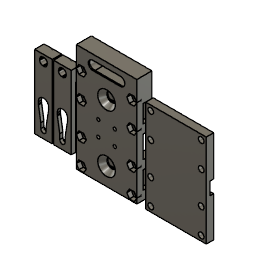
tool change neck (Autodesk Fusion 360 design; units mm, degrees)
Autodesk Fusion 360 part; units mm, degrees
note: some values were not read from the file. Set by a fixed rule: which sketch regions a step uses.
sketch "Sketch1" plane through (0, 0, 0) normal (0, 0, 1) x (1, 0, 0)
  line L0 (24, 8.75) -> (-24, 8.75)
  line L1 (-24, 8.75) -> (-24, -8.75)
  line L2 (-24, -8.75) -> (24, -8.75)
  line L3 (24, -8.75) -> (24, 8.75)
  line L4 (24, 8.75) -> (-24, -8.75) construction
  line L5 (-24, 8.75) -> (24, -8.75) construction
  line L6 (6.5, 6) -> (-6.5, 6)
  line L7 (-6.5, 6) -> (-6.5, -6)
  line L8 (-6.5, -6) -> (6.5, -6)
  line L9 (6.5, -6) -> (6.5, 6)
  line L10 (6.5, 6) -> (-6.5, -6) construction
  line L11 (-6.5, 6) -> (6.5, -6) construction
  circle A0 centre (6.5, 6) radius 1.25
  circle A1 centre (6.5, -6) radius 1.25
  circle A2 centre (-6.5, -6) radius 1.25
  circle A3 centre (-6.5, 6) radius 1.25
  line L12 (24, 36.75) -> (-24, 36.75)
  line L13 (-24, 36.75) -> (-24, -36.75)
  line L14 (-24, -36.75) -> (24, -36.75)
  line L15 (24, -36.75) -> (24, 36.75)
  line L16 (24, 36.75) -> (-24, -36.75) construction
  line L17 (-24, 36.75) -> (24, -36.75) construction
  circle A4 centre (6.5, 6) radius 3
  circle A5 centre (6.5, -6) radius 3
  circle A6 centre (-6.5, -6) radius 3
  circle A7 centre (-6.5, 6) radius 3
  line L18 (0, 36.75) -> (0, 22.75)
  circle A8 centre (0, 22.75) radius 4
  line L19 (0, -36.75) -> (0, -22.75)
  circle A9 centre (0, -22.75) radius 4
  line L20 (24, 36.75) -> (20, 36.75)
  line L21 (20, 36.75) -> (20, 32.75)
  line L22 (20, 32.75) -> (24, 32.75)
  line L23 (24, 32.75) -> (24, 36.75)
  line L24 (-24, 36.75) -> (-20, 36.75)
  line L25 (-20, 36.75) -> (-20, 32.75)
  line L26 (-20, 32.75) -> (-24, 32.75)
  line L27 (-24, 32.75) -> (-24, 36.75)
  line L28 (24, -36.75) -> (20, -36.75)
  line L29 (20, -36.75) -> (20, -32.75)
  line L30 (20, -32.75) -> (24, -32.75)
  line L31 (24, -32.75) -> (24, -36.75)
  line L32 (-24, -36.75) -> (-20, -36.75)
  line L33 (-20, -36.75) -> (-20, -32.75)
  line L34 (-20, -32.75) -> (-24, -32.75)
  line L35 (-24, -32.75) -> (-24, -36.75)
  circle A10 centre (-20, -32.75) radius 0.95
  circle A11 centre (20, -32.75) radius 0.95
  circle A12 centre (20, 32.75) radius 0.95
  circle A13 centre (-20, 32.75) radius 0.95
  circle A14 centre (-20, 32.75) radius 1.85
  circle A15 centre (20, 32.75) radius 1.85
  circle A16 centre (-20, -32.75) radius 1.85
  circle A17 centre (20, -32.75) radius 1.85
  line L36 (24, 8.75) -> (20, 8.75)
  line L37 (20, 8.75) -> (20, 12.75)
  line L38 (20, 12.75) -> (24, 12.75)
  line L39 (24, 12.75) -> (24, 8.75)
  line L40 (-24, 8.75) -> (-20, 8.75)
  line L41 (-20, 8.75) -> (-20, 12.75)
  line L42 (-20, 12.75) -> (-24, 12.75)
  line L43 (-24, 12.75) -> (-24, 8.75)
  line L44 (-24, -8.75) -> (-20, -8.75)
  line L45 (-20, -8.75) -> (-20, -12.75)
  line L46 (-20, -12.75) -> (-24, -12.75)
  line L47 (-24, -12.75) -> (-24, -8.75)
  line L48 (24, -8.75) -> (20, -8.75)
  line L49 (20, -8.75) -> (20, -12.75)
  line L50 (20, -12.75) -> (24, -12.75)
  line L51 (24, -12.75) -> (24, -8.75)
  circle A18 centre (-20, -12.75) radius 1.85
  circle A19 centre (20, -12.75) radius 1.85
  circle A20 centre (-20, 12.75) radius 1.85
  circle A21 centre (20, 12.75) radius 1.85
  line L52 (-24, 36.75) -> (-24, 22.75)
  line L53 (-24, 22.75) -> (-4, 22.75)
  line L54 (-24, -36.75) -> (-24, -22.75)
  line L55 (-24, -22.75) -> (-4, -22.75)
  circle A22 centre (-14, -22.75) radius 1.9
  circle A23 centre (-14, 22.75) radius 1.9
  line L56 (99, -36.75) -> (51, -36.75)
  line L57 (51, -36.75) -> (51, 36.75)
  line L58 (51, 36.75) -> (99, 36.75)
  line L59 (99, 36.75) -> (99, -36.75)
  line L60 (99, -36.75) -> (51, 36.75) construction
  line L61 (51, -36.75) -> (99, 36.75) construction
  line L62 (99, -8.75) -> (51, -8.75)
  line L63 (51, -8.75) -> (51, 8.75)
  line L64 (51, 8.75) -> (99, 8.75)
  line L65 (99, 8.75) -> (99, -8.75)
  line L66 (99, -8.75) -> (51, 8.75) construction
  line L67 (51, -8.75) -> (99, 8.75) construction
  line L68 (51, 36.75) -> (55, 36.75)
  line L69 (55, 36.75) -> (55, 32.75)
  line L70 (55, 32.75) -> (51, 32.75)
  line L71 (51, 32.75) -> (51, 36.75)
  line L72 (99, 36.75) -> (95, 36.75)
  line L73 (95, 36.75) -> (95, 32.75)
  line L74 (95, 32.75) -> (99, 32.75)
  line L75 (99, 32.75) -> (99, 36.75)
  line L76 (51, -36.75) -> (55, -36.75)
  line L77 (55, -36.75) -> (55, -32.75)
  line L78 (55, -32.75) -> (51, -32.75)
  line L79 (51, -32.75) -> (51, -36.75)
  line L80 (99, -36.75) -> (95, -36.75)
  line L81 (95, -36.75) -> (95, -32.75)
  line L82 (95, -32.75) -> (99, -32.75)
  line L83 (99, -32.75) -> (99, -36.75)
  circle A24 centre (55, 32.75) radius 2.25
  circle A25 centre (95, 32.75) radius 2.25
  circle A26 centre (55, -32.75) radius 2.25
  circle A27 centre (95, -32.75) radius 2.25
  line L84 (51, 8.75) -> (55, 8.75)
  line L85 (55, 8.75) -> (55, 12.75)
  line L86 (55, 12.75) -> (51, 12.75)
  line L87 (51, 12.75) -> (51, 8.75)
  circle A28 centre (55, 12.75) radius 2.25
  line L88 (99, 8.75) -> (95, 8.75)
  line L89 (95, 8.75) -> (95, 12.75)
  line L90 (95, 12.75) -> (99, 12.75)
  line L91 (99, 12.75) -> (99, 8.75)
  circle A29 centre (95, 12.75) radius 2.25
  line L92 (51, -8.75) -> (55, -8.75)
  line L93 (55, -8.75) -> (55, -12.75)
  line L94 (55, -12.75) -> (51, -12.75)
  line L95 (51, -12.75) -> (51, -8.75)
  line L96 (99, -8.75) -> (95, -8.75)
  line L97 (95, -8.75) -> (95, -12.75)
  line L98 (95, -12.75) -> (99, -12.75)
  line L99 (99, -12.75) -> (99, -8.75)
  circle A30 centre (55, -12.75) radius 2.25
  circle A31 centre (95, -12.75) radius 2.25
  line L100 (99, 5) -> (51, 5)
  line L101 (51, 5) -> (51, -5)
  line L102 (51, -5) -> (99, -5)
  line L103 (99, -5) -> (99, 5)
  line L104 (99, 5) -> (51, -5) construction
  line L105 (51, 5) -> (99, -5) construction
  line L106 (-43, -29) -> (-57, -29)
  line L107 (-57, -29) -> (-57, 29)
  line L108 (-57, 29) -> (-43, 29)
  line L109 (-43, 29) -> (-43, -29)
  line L110 (-43, -29) -> (-57, 29) construction
  line L111 (-57, -29) -> (-43, 29) construction
  line L112 (-57, 29) -> (-43, 29)
  line L113 (-43, 29) -> (-43, 19)
  line L114 (-43, 19) -> (-57, 19)
  line L115 (-57, 19) -> (-57, 29)
  line L116 (-43, 19) -> (-43, 21.5068)
  line L117 (-43, 21.5068) -> (-43, 29)
  line L118 (-44, 29) -> (-44, 29)
  line L119 (-43, 29) -> (-43, 19)
  line L120 (-43, 29) -> (-50, 29)
  line L121 (-50, 29) -> (-50, 24)
  line L122 (-50, 24) -> (-43, 24)
  line L123 (-43, 24) -> (-43, 29)
  line L124 (-47, 27) -> (-53, 27)
  line L125 (-53, 27) -> (-53, 21)
  line L126 (-53, 21) -> (-47, 21)
  line L127 (-47, 21) -> (-47, 27)
  line L128 (-47, 27) -> (-53, 21) construction
  line L129 (-53, 27) -> (-47, 21) construction
  line L130 (-50, 24) -> (-50, -5)
  circle A32 centre (-50, -5) radius 4
  line L131 (-50, -5) -> (-50, -7)
  line L132 (-50, -7) -> (-50, -19)
  circle A33 centre (-50, -7) radius 4
  line L133 (-46.0119, -4.6913) -> (-46.0001, -6.9792)
  line L134 (-53.9727, -5.4669) -> (-53.9993, -6.9269)
  circle A34 centre (-50, -19) radius 2.1
  line L135 (-50, -19) -> (-50, -23)
  circle A35 centre (-50, -23) radius 2.1
  line L136 (-47.9, -19) -> (-47.9, -23)
  line L137 (-52.1, -23) -> (-52.1, -19)
  line L138 (-47.9, -19) -> (-46.0519, -7.6424)
  line L139 (-52.1, -19) -> (-53.9481, -7.6424)
  line L140 (-24, 36.75) -> (24, 36.75)
  line L141 (24, 36.75) -> (24, 46.75)
  line L142 (24, 46.75) -> (-24, 46.75)
  line L143 (-24, 46.75) -> (-24, 36.75)
  line L144 (51, 36.75) -> (99, 36.75)
  line L145 (99, 36.75) -> (99, 46.75)
  line L146 (99, 46.75) -> (51, 46.75)
  line L147 (51, 46.75) -> (51, 36.75)
  line L148 (51, 46.75) -> (55, 46.75)
  line L149 (55, 46.75) -> (55, 42.75)
  line L150 (55, 42.75) -> (51, 42.75)
  line L151 (51, 42.75) -> (51, 46.75)
  line L152 (99, 46.75) -> (95, 46.75)
  line L153 (95, 46.75) -> (95, 42.75)
  line L154 (95, 42.75) -> (99, 42.75)
  line L155 (99, 42.75) -> (99, 46.75)
  circle A36 centre (95, 42.75) radius 2.25
  circle A37 centre (55, 42.75) radius 2.25
  line L156 (24, 46.75) -> (20, 46.75)
  line L157 (20, 46.75) -> (20, 42.75)
  line L158 (20, 42.75) -> (24, 42.75)
  line L159 (24, 42.75) -> (24, 46.75)
  line L160 (-24, 46.75) -> (-20, 46.75)
  line L161 (-20, 46.75) -> (-20, 42.75)
  line L162 (-20, 42.75) -> (-24, 42.75)
  line L163 (-24, 42.75) -> (-24, 46.75)
  circle A38 centre (20, 42.75) radius 1.85
  circle A39 centre (-20, 42.75) radius 1.85
  line L164 (21.963, 29.35) -> (23.926, 32.75)
  line L165 (23.926, 32.75) -> (21.963, 36.15)
  line L166 (21.963, 36.15) -> (18.037, 36.15)
  line L167 (18.037, 36.15) -> (16.074, 32.75)
  line L168 (16.074, 32.75) -> (18.037, 29.35)
  line L169 (18.037, 29.35) -> (21.963, 29.35)
  line L170 (-18.037, 29.35) -> (-16.074, 32.75)
  line L171 (-16.074, 32.75) -> (-18.037, 36.15)
  line L172 (-18.037, 36.15) -> (-21.963, 36.15)
  line L173 (-21.963, 36.15) -> (-23.926, 32.75)
  line L174 (-23.926, 32.75) -> (-21.963, 29.35)
  line L175 (-21.963, 29.35) -> (-18.037, 29.35)
  line L176 (21.963, -36.15) -> (23.926, -32.75)
  line L177 (23.926, -32.75) -> (21.963, -29.35)
  line L178 (21.963, -29.35) -> (18.037, -29.35)
  line L179 (18.037, -29.35) -> (16.074, -32.75)
  line L180 (16.074, -32.75) -> (18.037, -36.15)
  line L181 (18.037, -36.15) -> (21.963, -36.15)
  line L182 (-18.037, -36.15) -> (-16.074, -32.75)
  line L183 (-16.074, -32.75) -> (-18.037, -29.35)
  line L184 (-18.037, -29.35) -> (-21.963, -29.35)
  line L185 (-21.963, -29.35) -> (-23.926, -32.75)
  line L186 (-23.926, -32.75) -> (-21.963, -36.15)
  line L187 (-21.963, -36.15) -> (-18.037, -36.15)
  line L188 (21.963, 9.35) -> (23.926, 12.75)
  line L189 (23.926, 12.75) -> (21.963, 16.15)
  line L190 (21.963, 16.15) -> (18.037, 16.15)
  line L191 (18.037, 16.15) -> (16.074, 12.75)
  line L192 (16.074, 12.75) -> (18.037, 9.35)
  line L193 (18.037, 9.35) -> (21.963, 9.35)
  line L194 (21.963, -16.15) -> (23.926, -12.75)
  line L195 (23.926, -12.75) -> (21.963, -9.35)
  line L196 (21.963, -9.35) -> (18.037, -9.35)
  line L197 (18.037, -9.35) -> (16.074, -12.75)
  line L198 (16.074, -12.75) -> (18.037, -16.15)
  line L199 (18.037, -16.15) -> (21.963, -16.15)
  line L200 (-18.037, 9.35) -> (-16.074, 12.75)
  line L201 (-16.074, 12.75) -> (-18.037, 16.15)
  line L202 (-18.037, 16.15) -> (-21.963, 16.15)
  line L203 (-21.963, 16.15) -> (-23.926, 12.75)
  line L204 (-23.926, 12.75) -> (-21.963, 9.35)
  line L205 (-21.963, 9.35) -> (-18.037, 9.35)
  line L206 (-18.037, -16.15) -> (-16.074, -12.75)
  line L207 (-16.074, -12.75) -> (-18.037, -9.35)
  line L208 (-18.037, -9.35) -> (-21.963, -9.35)
  line L209 (-21.963, -9.35) -> (-23.926, -12.75)
  line L210 (-23.926, -12.75) -> (-21.963, -16.15)
  line L211 (-21.963, -16.15) -> (-18.037, -16.15)
  point P0 (75, 0)
  point P1 (75, 0)
  point P2 (75, 0)
  point P3 (-50, 0)
  point P4 (-50, 24)
  point P5 (20, 32.75)
  point P6 (-20, 32.75)
  point P7 (20, -32.75)
  point P8 (-20, -32.75)
  point P9 (20, 12.75)
  point P10 (20, -12.75)
  point P11 (-20, 12.75)
  point P12 (-20, -12.75)
  dimension "d1" = 48
  dimension "d2" = 17.5
  dimension "d3" = 13
  dimension "d4" = 12
  dimension "d5" = 2.5
  dimension "d6" = 2.5
  dimension "d7" = 2.5
  dimension "d8" = 2.5
  dimension "d11" = 48
  dimension "d12" = 73.5
  dimension "d30" = 6
  dimension "d31" = 6
  dimension "d32" = 6
  dimension "d33" = 6
  dimension "d38" = 14
  dimension "d39" = 8
  dimension "d40" = 14
  dimension "d41" = 8
  dimension "d50" = 4
  dimension "d51" = 4
  dimension "d52" = 4
  dimension "d53" = 4
  dimension "d54" = 4
  dimension "d55" = 4
  dimension "d56" = 4
  dimension "d57" = 4
  dimension "d58" = 1.9
  dimension "d59" = 1.9
  dimension "d60" = 1.9
  dimension "d61" = 1.9
  dimension "d62" = 3.7
  dimension "d63" = 3.7
  dimension "d64" = 3.7
  dimension "d65" = 3.7
  dimension "d86" = 4
  dimension "d87" = 4
  dimension "d88" = 4
  dimension "d89" = 4
  dimension "d90" = 4
  dimension "d91" = 4
  dimension "d92" = 4
  dimension "d93" = 4
  dimension "d94" = 3.7
  dimension "d95" = 3.7
  dimension "d96" = 3.7
  dimension "d97" = 3.7
  dimension "d114" = 14
  dimension "d115" = 14
  dimension "d116" = 3.8
  dimension "d117" = 3.8
  dimension "d118" = 48
  dimension "d119" = 73.5
  dimension "d120" = 48
  dimension "d121" = 17.5
  dimension "d122" = 4
  dimension "d123" = 4
  dimension "d124" = 4
  dimension "d125" = 4
  dimension "d126" = 4
  dimension "d127" = 4
  dimension "d128" = 4
  dimension "d129" = 4
  dimension "d130" = 4.5
  dimension "d131" = 4.5
  dimension "d132" = 4.5
  dimension "d133" = 4.5
  dimension "d136" = 4
  dimension "d137" = 4
  dimension "d138" = 4.5
  dimension "d139" = 4
  dimension "d140" = 4
  dimension "d141" = 4.5
  dimension "d142" = 4
  dimension "d143" = 4
  dimension "d144" = 4
  dimension "d145" = 4
  dimension "d146" = 4.5
  dimension "d147" = 4.5
  dimension "d148" = 48
  dimension "d149" = 10
  dimension "d154" = 14
  dimension "d155" = 58
  dimension "d156" = 14
  dimension "d157" = 10
  dimension "d158" = 7
  dimension "d159" = 5
  dimension "d160" = 6
  dimension "d161" = 6
  dimension "d162" = 29
  dimension "d163" = 8
  dimension "d164" = 2
  dimension "d165" = 12
  dimension "d166" = 8
  dimension "d167" = 4.2
  dimension "d168" = 4
  dimension "d169" = 4.2
  dimension "d211" = 10
  dimension "d212" = 48
  dimension "d213" = 10
  dimension "d214" = 4
  dimension "d215" = 4
  dimension "d216" = 4
  dimension "d217" = 4
  dimension "d218" = 4.5
  dimension "d219" = 4.5
  dimension "d220" = 4
  dimension "d221" = 4
  dimension "d222" = 4
  dimension "d223" = 4
  dimension "d224" = 3.7
  dimension "d225" = 3.7
  dimension "d254" = 3.4
  dimension "d255" = 3.4
  dimension "d256" = 3.4
  dimension "d257" = 3.4
  dimension "d262" = 3.4
  dimension "d263" = 3.4
  dimension "d264" = 3.4
  dimension "d265" = 3.4
  constraint horizontal L0
  constraint perpendicular L0 L1
  constraint parallel L0 L2
  constraint parallel L1 L3
  constraint coincident L4 origin
  constraint coincident L5 origin
  constraint horizontal L6
  constraint perpendicular L6 L7
  constraint parallel L6 L8
  constraint parallel L7 L9
  constraint coincident L10 origin
  constraint coincident L11 origin
  constraint coincident L6.start L9.end
  constraint coincident L8.end L9.start
  constraint coincident L7.end L8.start
  constraint coincident L6.end L7.start
  constraint horizontal L12
  constraint perpendicular L12 L13
  constraint parallel L12 L14
  constraint parallel L13 L15
  constraint coincident L16 origin
  constraint coincident L17 origin
  constraint concentric A0 A4
  constraint concentric A1 A5
  constraint concentric A2 A6
  constraint concentric A3 A7
  constraint midpoint L12 L18.start
  constraint perpendicular L12 L18
  constraint coincident L18.end A8.centre
  constraint midpoint L14 L19.start
  constraint perpendicular L14 L19
  constraint coincident L19.end A9.centre
  constraint horizontal L20
  constraint vertical L21
  constraint horizontal L22
  constraint vertical L23
  constraint horizontal L24
  constraint vertical L25
  constraint horizontal L26
  constraint vertical L27
  constraint horizontal L28
  constraint vertical L29
  constraint horizontal L30
  constraint vertical L31
  constraint horizontal L32
  constraint vertical L33
  constraint horizontal L34
  constraint vertical L35
  constraint coincident P8 L33.end
  constraint coincident P7 L29.end
  constraint coincident P5 L21.end
  constraint coincident P6 L25.end
  constraint concentric A13 A14
  constraint concentric A10 A16
  constraint concentric A11 A17
  constraint horizontal L36
  constraint vertical L37
  constraint horizontal L38
  constraint vertical L39
  constraint horizontal L40
  constraint vertical L41
  constraint horizontal L42
  constraint vertical L43
  constraint horizontal L44
  constraint vertical L45
  constraint horizontal L46
  constraint vertical L47
  constraint horizontal L48
  constraint vertical L49
  constraint horizontal L50
  constraint vertical L51
  constraint coincident P12 L45.end
  constraint coincident P10 L49.end
  constraint coincident P11 L41.end
  constraint coincident P9 L37.end
  constraint perpendicular L26 L52
  constraint coincident A8 L53.end
  constraint perpendicular L52 L53
  constraint perpendicular L14 L54
  constraint coincident A9 L55.end
  constraint perpendicular L54 L55
  constraint midpoint L55 A22.centre
  constraint midpoint L53 A23.centre
  constraint horizontal L56
  constraint perpendicular L56 L57
  constraint parallel L56 L58
  constraint parallel L57 L59
  constraint coincident L60 P2
  constraint coincident L61 P2
  constraint horizontal L62
  constraint perpendicular L62 L63
  constraint parallel L62 L64
  constraint parallel L63 L65
  constraint coincident L66 P2
  constraint coincident L67 P2
  constraint coincident P2 P1
  constraint horizontal L68
  constraint vertical L69
  constraint horizontal L70
  constraint vertical L71
  constraint horizontal L72
  constraint vertical L73
  constraint horizontal L74
  constraint vertical L75
  constraint horizontal L76
  constraint vertical L77
  constraint horizontal L78
  constraint vertical L79
  constraint horizontal L80
  constraint vertical L81
  constraint horizontal L82
  constraint vertical L83
  constraint coincident L69.end L70.start
  constraint coincident L73.end L74.start
  constraint coincident L77.end L78.start
  constraint coincident L81.end L82.start
  constraint horizontal L84
  constraint vertical L85
  constraint horizontal L86
  constraint vertical L87
  constraint coincident L85.end L86.start
  constraint horizontal L88
  constraint vertical L89
  constraint horizontal L90
  constraint vertical L91
  constraint coincident L89.end L90.start
  constraint horizontal L92
  constraint vertical L93
  constraint horizontal L94
  constraint vertical L95
  constraint horizontal L96
  constraint vertical L97
  constraint horizontal L98
  constraint vertical L99
  constraint coincident L93.end L94.start
  constraint coincident L97.end L98.start
  constraint horizontal L100
  constraint perpendicular L100 L101
  constraint parallel L100 L102
  constraint parallel L101 L103
  constraint coincident L104 P2
  constraint coincident L105 P2
  constraint horizontal L106
  constraint perpendicular L106 L107
  constraint parallel L106 L108
  constraint parallel L107 L109
  constraint coincident L110 P3
  constraint coincident L111 P3
  constraint horizontal L112
  constraint vertical L113
  constraint horizontal L114
  constraint vertical L115
  constraint vertical L117
  constraint vertical L119
  constraint coincident L113 L108.end
  constraint horizontal L120
  constraint vertical L121
  constraint horizontal L122
  constraint vertical L123
  constraint horizontal L124
  constraint perpendicular L124 L125
  constraint parallel L124 L126
  constraint parallel L125 L127
  constraint coincident L128 P4
  constraint coincident L129 P4
  constraint coincident P4 L121.end
  constraint perpendicular L114 L130
  constraint coincident L130.end A32.centre
  constraint vertical L131
  constraint parallel L131 L132
  constraint coincident L131.end L132.start
  constraint coincident A32 L133.start
  constraint coincident A33 L133.end
  constraint tangent A33 L133
  constraint coincident A32 L134.start
  constraint coincident A33 L134.end
  constraint tangent A33 L134
  constraint coincident L132.end A34.centre
  constraint parallel L132 L135
  constraint coincident L135.end A35.centre
  constraint coincident A34 L136.start
  constraint coincident A35 L136.end
  constraint tangent A35 L136
  constraint parallel L132 L136
  constraint coincident A35 L137.start
  constraint coincident A34 L137.end
  constraint tangent A34 L137
  constraint vertical L137
  constraint coincident A33 L138.end
  constraint tangent A33 L138
  constraint coincident A33 L139.end
  constraint tangent A33 L139
  constraint horizontal L140
  constraint vertical L141
  constraint horizontal L142
  constraint vertical L143
  constraint horizontal L144
  constraint vertical L145
  constraint horizontal L146
  constraint vertical L147
  constraint horizontal L148
  constraint vertical L149
  constraint horizontal L150
  constraint vertical L151
  constraint horizontal L152
  constraint vertical L153
  constraint horizontal L154
  constraint vertical L155
  constraint coincident L153.end L154.start
  constraint coincident L149.end L150.start
  constraint horizontal L156
  constraint vertical L157
  constraint horizontal L158
  constraint vertical L159
  constraint horizontal L160
  constraint vertical L161
  constraint horizontal L162
  constraint vertical L163
  constraint coincident L157.end L158.start
  constraint coincident L161.end L162.start
  measures "d1" distance of L1.end L2.end
  measures "d2" distance of L0.end L1.end
  measures "d3" distance of L7.end L8.end
  measures "d4" distance of L6.end L7.end
  measures "d5" diameter of A0
  measures "d6" diameter of A1
  measures "d7" diameter of A2
  measures "d8" diameter of A3
  measures "d11" distance of L13.end L14.end
  measures "d12" distance of L12.end L13.end
  measures "d30" diameter of A4
  measures "d31" diameter of A5
  measures "d32" diameter of A6
  measures "d33" diameter of A7
  measures "d38" distance of L18.start L18.end
  measures "d39" diameter of A8
  measures "d40" distance of L19.start L19.end
  measures "d41" diameter of A9
  measures "d50" distance of L12.start L20.end
  measures "d51" distance of L12.start L22.end
  measures "d52" distance of L12.end L24.end
  measures "d53" distance of L12.end L26.end
  measures "d54" distance of L14.end L28.end
  measures "d55" distance of L14.end L30.end
  measures "d56" distance of L13.end L32.end
  measures "d57" distance of L13.end L34.end
  measures "d58" diameter of A10
  measures "d59" diameter of A11
  measures "d60" diameter of A12
  measures "d61" diameter of A13
  measures "d62" diameter of A14
  measures "d63" diameter of A15
  measures "d64" diameter of A16
  measures "d65" diameter of A17
  measures "d86" distance of L0.start L36.end
  measures "d87" distance of L0.start L38.end
  measures "d88" distance of L0.end L40.end
  measures "d89" distance of L0.end L42.end
  measures "d90" distance of L1.end L44.end
  measures "d91" distance of L1.end L46.end
  measures "d92" distance of L2.end L48.end
  measures "d93" distance of L2.end L50.end
  measures "d94" diameter of A18
  measures "d95" diameter of A19
  measures "d96" diameter of A20
  measures "d97" diameter of A21
  measures "d114" distance of L12.end L52.end
  measures "d115" distance of L13.end L54.end
  measures "d116" diameter of A22
  measures "d117" diameter of A23
  measures "d118" distance of L57.end L58.end
  measures "d119" distance of L56.end L57.end
  measures "d120" distance of L63.end L64.end
  measures "d121" distance of L62.end L63.end
  measures "d122" distance of L57.end L68.end
  measures "d123" distance of L57.end L70.end
  measures "d124" distance of L58.end L72.end
  measures "d125" distance of L58.end L74.end
  measures "d126" distance of L56.end L76.end
  measures "d127" distance of L56.end L78.end
  measures "d128" distance of L56.start L80.end
  measures "d129" distance of L56.start L82.end
  measures "d130" diameter of A24
  measures "d131" diameter of A25
  measures "d132" diameter of A26
  measures "d133" diameter of A27
  measures "d136" distance of L63.end L84.end
  measures "d137" distance of L63.end L86.end
  measures "d138" diameter of A28 A4
  measures "d139" distance of L64.end L88.end
  measures "d140" distance of L64.end L90.end
  measures "d141" diameter of A29
  measures "d142" distance of L62.end L92.end
  measures "d143" distance of L62.end L94.end
  measures "d144" distance of L62.start L96.end
  measures "d145" distance of L62.start L98.end
  measures "d146" diameter of A30
  measures "d147" diameter of A31
  measures "d148" distance of L101.end L102.end
  measures "d149" distance of L100.end L101.end
  measures "d154" distance of L107.end L108.end
  measures "d155" distance of L106.end L107.end
  measures "d156" distance of L107.end L108.end
  measures "d157" distance of L107.end L114.end
  measures "d158" distance of L108.end L120.end
  measures "d159" distance of L108.end L122.end
  measures "d160" distance of L125.end L126.end
  measures "d161" distance of L124.end L125.end
  measures "d162" distance of P4 L130.end
  measures "d163" diameter of A32
  measures "d164" distance of L130.end L131.end
  measures "d165" distance of L131.end L132.end
  measures "d166" diameter of A33
  measures "d167" diameter of A34
  measures "d168" distance of L132.end L135.end
  measures "d169" diameter of A35
  measures "d211" distance of L12.end L142.end
  measures "d212" distance of L57.end L58.end
  measures "d213" distance of L57.end L146.end
  measures "d214" distance of L146.end L148.end
  measures "d215" distance of L146.end L150.end
  measures "d216" distance of L145.end L152.end
  measures "d217" distance of L145.end L154.end
  measures "d219" diameter of A37 A4
  measures "d220" distance of L141.end L156.end
  measures "d221" distance of L141.end L158.end
  measures "d222" distance of L142.end L160.end
  measures "d223" distance of L142.end L162.end
  measures "d224" diameter of A38
  measures "d225" diameter of A39
  measures "d254" distance of P5 L169
  measures "d255" distance of P6 L175
  measures "d256" distance of P7 L181
  measures "d257" distance of P8 L187
  measures "d262" distance of P9 L193
  measures "d263" distance of P10 L199
  measures "d264" distance of P11 L205
  measures "d265" distance of P12 L211
extrude "Extrude1" add sketch "Sketch1" along normal blind 12 contours L0 L2 L3 L9 L15 A4 A5 L36 L48 | L0 L15 L36 L37 L38 L39 L188 L193 | L0 L12 L13 L15 A4 A7 L18 A8 L21 L22 L37 L38 L41 L42 L53 A23 L140 L164 L166 L167 L168 L169 L189 L190 L191 L192 L193 L200 L201 L202 L203 L205 | L2 L15 L48 L49 L50 L51 L195 L196 | L0 L6 L9 A0 A4 | L0 A4 | L37 L38 A21 L189 L190 L191 L192 L193 | L37 L38 A21 L188 L193 | L2 L13 L14 L15 A5 A6 L19 A9 L29 L30 L45 L46 L49 L50 L55 A22 L177 L178 L179 L180 L181 L194 L196 L197 L198 L199 L206 L207 L208 L210 L211 | L12 L15 L20 L21 L22 L23 L140 L165 L166 | L0 L6 A4 A7 | L2 A5 | L2 L8 L9 A1 A5 | L49 L50 A19 L195 L196 | L49 L50 A19 L194 L196 L197 L198 L199 | L14 L15 L28 L29 L30 L31 L176 L181 | L21 L22 A15 L164 L166 L167 L168 L169 | L21 L22 A15 L165 L166 | L0 L6 L7 A3 A7 | L0 A7 | L6 L7 L8 L9 A4 A5 A6 A7 | L6 L9 A0 A4 | L2 L8 A5 A6 | L29 L30 A17 L176 L181 | L29 L30 A17 L177 L178 L179 L180 L181 | L0 L1 L2 L7 L13 A6 A7 L40 L44 | L6 L7 A3 A7 | L8 L9 A1 A5 | L2 A6 | L2 L7 L8 A2 A6 | L12 L13 L18 A8 L25 L26 L52 L53 A23 L140 L170 L171 L172 L174 L175 | L0 L13 L40 L41 L42 L43 L204 L205 | L7 L8 A2 A6 | L13 L14 L19 A9 L33 L34 L54 L55 A22 L182 L183 L184 L185 L187 | L12 L13 L24 L25 L26 L27 L52 L140 L172 L173 | A8 | L41 L42 A20 L204 L205 | L41 L42 A20 L200 L201 L202 L203 L205 | L2 L13 L44 L45 L46 L47 L208 L209 | L13 L14 L32 L33 L34 L35 L54 L186 L187 | A9 | L25 L26 A14 L170 L171 L172 L174 L175 | L25 L26 A14 L172 L173 | L45 L46 A18 L206 L207 L208 L210 L211 | L45 L46 A18 L208 L209 | L33 L34 A16 L186 L187 | L33 L34 A16 L182 L183 L184 L185 L187 | L53 A23 | L53 A23 | L55 A22 | L55 A22 makes body 1
extrude "Extrude2" cut sketch "Sketch1" along normal blind 7 contours L0 L2 L3 L9 L15 A4 A5 L36 L48 | L0 L6 L9 A0 A4 | L0 L6 A4 A7 | L2 L8 L9 A1 A5 | L0 L6 L7 A3 A7 | L6 L7 L8 L9 A4 A5 A6 A7 | L6 L9 A0 A4 | L2 L8 A5 A6 | L0 L1 L2 L7 L13 A6 A7 L40 L44 | L6 L7 A3 A7 | L8 L9 A1 A5 | L2 L7 L8 A2 A6 | L7 L8 A2 A6 bodies 1
extrude "Extrude3" cut sketch "Sketch1" along normal blind 19 contours A8 | A9 bodies 1
extrude "Extrude19" cut sketch "Sketch1" along normal blind 12 and the other way blind -8.5 contours L37 L38 A21 L189 L190 L191 L192 L193 | L37 L38 A21 L188 L193 | L49 L50 A19 L195 L196 | L49 L50 A19 L194 L196 L197 L198 L199 | L21 L22 A15 L164 L166 L167 L168 L169 | L21 L22 A15 L165 L166 | L29 L30 A17 L176 L181 | L29 L30 A17 L177 L178 L179 L180 L181 | L41 L42 A20 L204 L205 | L41 L42 A20 L200 L201 L202 L203 L205 | L25 L26 A14 L170 L171 L172 L174 L175 | L25 L26 A14 L172 L173 | L45 L46 A18 L206 L207 L208 L210 L211 | L45 L46 A18 L208 L209 | L33 L34 A16 L186 L187 | L33 L34 A16 L182 L183 L184 L185 L187 bodies 1
sketch "Sketch3" plane through (24, 0, 0) normal (1, 0, 0) x (0, 0, -1)
  line L0 (0, 8.75) -> (0, 36.75)
  line L1 (-12, 36.75) -> (-12, -36.75)
  line L2 (-12, -36.75) -> (0, -36.75)
  line L3 (-12, 36.75) -> (-7, 36.75)
  line L4 (-7, 36.75) -> (-7, -36.75)
  line L5 (-7, -36.75) -> (-12, -36.75)
  line L6 (-12, -36.75) -> (-12, 36.75)
  line L7 (-7, 36.75) -> (-7, 28.75)
  line L8 (-7, 28.75) -> (-3, 28.75)
  line L9 (-3, 28.75) -> (-3, 16.75)
  line L10 (-3, 16.75) -> (-7, 16.75)
  line L11 (-7, 16.75) -> (-7, 28.75)
  line L12 (-7, -36.75) -> (-7, -28.75)
  line L13 (-7, -28.75) -> (-3, -28.75)
  line L14 (-3, -28.75) -> (-3, -16.75)
  line L15 (-3, -16.75) -> (-7, -16.75)
  line L16 (-7, -16.75) -> (-7, -28.75)
  line L17 (-7, 12.75) -> (-7, 28.75)
  line L18 (-7, -24.75) -> (-7, -16.75)
  line L19 (-7, -24.75) -> (-7, -23.75)
  line L20 (-7, 28.75) -> (-10, 28.75)
  line L21 (-10, 28.75) -> (-10, 16.75)
  line L22 (-10, 16.75) -> (-7, 16.75)
  line L23 (-7, 16.75) -> (-7, 28.75)
  line L24 (-7, 28.75) -> (-9, 28.75)
  line L25 (-9, 28.75) -> (-9, 16.75)
  line L26 (-9, 16.75) -> (-7, 16.75)
  line L27 (-7, 16.75) -> (-7, 28.75)
  line L28 (-9, 28.75) -> (-7, 28.75)
  line L29 (-7, 28.75) -> (-7, 27.75)
  line L30 (-7, 27.75) -> (-9, 27.75)
  line L31 (-9, 27.75) -> (-9, 28.75)
  line L32 (-7, 16.75) -> (-9, 16.75)
  line L33 (-9, 16.75) -> (-9, 17.75)
  line L34 (-9, 17.75) -> (-7, 17.75)
  line L35 (-7, 17.75) -> (-7, 16.75)
  line L36 (-7, -16.75) -> (-10, -16.75)
  line L37 (-10, -16.75) -> (-10, -28.75)
  line L38 (-10, -28.75) -> (-7, -28.75)
  line L39 (-7, -28.75) -> (-7, -16.75)
  line L40 (-7, -16.75) -> (-9, -16.75)
  line L41 (-9, -16.75) -> (-9, -28.75)
  line L42 (-9, -28.75) -> (-7, -28.75)
  line L43 (-7, -28.75) -> (-7, -16.75)
  line L44 (-7, -16.75) -> (-9, -16.75)
  line L45 (-9, -16.75) -> (-9, -17.75)
  line L46 (-9, -17.75) -> (-7, -17.75)
  line L47 (-7, -17.75) -> (-7, -16.75)
  line L48 (-7, -28.75) -> (-9, -28.75)
  line L49 (-9, -28.75) -> (-9, -27.75)
  line L50 (-9, -27.75) -> (-7, -27.75)
  line L51 (-7, -27.75) -> (-7, -28.75)
  line L52 (-3, 28.75) -> (-7, 28.75)
  line L53 (-7, 28.75) -> (-7, 29.75)
  line L54 (-7, 29.75) -> (-3, 29.75)
  line L55 (-3, 29.75) -> (-3, 28.75)
  line L56 (-3, 16.75) -> (-7, 16.75)
  line L57 (-7, 16.75) -> (-7, 15.75)
  line L58 (-7, 15.75) -> (-3, 15.75)
  line L59 (-3, 15.75) -> (-3, 16.75)
  line L60 (-3, -16.75) -> (-7, -16.75)
  line L61 (-7, -16.75) -> (-7, -15.75)
  line L62 (-7, -15.75) -> (-3, -15.75)
  line L63 (-3, -15.75) -> (-3, -16.75)
  line L64 (-3, -28.75) -> (-7, -28.75)
  line L65 (-7, -28.75) -> (-7, -29.75)
  line L66 (-7, -29.75) -> (-3, -29.75)
  line L67 (-3, -29.75) -> (-3, -28.75)
  line L68 (0, 36.75) -> (-12, 36.75)
  line L69 (-7, 8.75) -> (0, 8.75)
  line L70 (0, -36.75) -> (0, -8.75)
  line L71 (0, -8.75) -> (-7, -8.75)
  line L72 (-7, -8.75) -> (-7, 8.75)
  dimension "d42" = 5
  dimension "d43" = 73.5
  dimension "d44" = 8
  dimension "d45" = 4
  dimension "d46" = 12
  dimension "d47" = 8
  dimension "d48" = 4
  dimension "d49" = 12
  dimension "d98" = 3
  dimension "d99" = 12
  dimension "d100" = 2
  dimension "d101" = 12
  dimension "d102" = 2
  dimension "d103" = 1
  dimension "d104" = 2
  dimension "d105" = 1
  dimension "d106" = 3
  dimension "d107" = 12
  dimension "d108" = 2
  dimension "d109" = 12
  dimension "d110" = 2
  dimension "d111" = 1
  dimension "d112" = 2
  dimension "d113" = 1
  dimension "d226" = 4
  dimension "d227" = 1
  dimension "d228" = 4
  dimension "d229" = 1
  dimension "d230" = 4
  dimension "d231" = 1
  dimension "d232" = 4
  dimension "d233" = 1
  constraint horizontal L3
  constraint vertical L4
  constraint horizontal L5
  constraint vertical L6
  constraint coincident L1.start L3.start
  constraint perpendicular L3 L7
  constraint horizontal L8
  constraint vertical L9
  constraint horizontal L10
  constraint vertical L11
  constraint perpendicular L5 L12
  constraint horizontal L13
  constraint vertical L14
  constraint horizontal L15
  constraint vertical L16
  constraint vertical L17
  constraint vertical L18
  constraint horizontal L20
  constraint vertical L21
  constraint horizontal L22
  constraint vertical L23
  constraint horizontal L24
  constraint vertical L25
  constraint horizontal L26
  constraint vertical L27
  constraint horizontal L28
  constraint vertical L29
  constraint horizontal L30
  constraint vertical L31
  constraint horizontal L32
  constraint vertical L33
  constraint horizontal L34
  constraint vertical L35
  constraint horizontal L36
  constraint vertical L37
  constraint horizontal L38
  constraint vertical L39
  constraint horizontal L40
  constraint vertical L41
  constraint horizontal L42
  constraint vertical L43
  constraint horizontal L44
  constraint vertical L45
  constraint horizontal L46
  constraint vertical L47
  constraint horizontal L48
  constraint vertical L49
  constraint horizontal L50
  constraint vertical L51
  constraint horizontal L52
  constraint vertical L53
  constraint horizontal L54
  constraint vertical L55
  constraint horizontal L56
  constraint vertical L57
  constraint horizontal L58
  constraint vertical L59
  constraint horizontal L60
  constraint vertical L61
  constraint horizontal L62
  constraint vertical L63
  constraint horizontal L64
  constraint vertical L65
  constraint horizontal L66
  constraint vertical L67
  measures "d42" distance of L1.start L3.end
  measures "d43" distance of L1.start L1.end
  measures "d44" distance of L3.end L7.end
  measures "d45" distance of L7.end L8.end
  measures "d46" distance of L7.end L10.end
  measures "d47" distance of L4.end L12.end
  measures "d48" distance of L12.end L13.end
  measures "d49" distance of L12.end L15.end
  measures "d98" distance of L7.end L20.end
  measures "d99" distance of L7.end L10.end
  measures "d100" distance of L7.end L24.end
  measures "d101" distance of L7.end L10.end
  measures "d102" distance of L24.end L7.end
  measures "d103" distance of L24.end L30.end
  measures "d104" distance of L10.end L25.end
  measures "d105" distance of L10.end L34.end
  measures "d106" distance of L15.end L36.end
  measures "d107" distance of L15.end L12.end
  measures "d108" distance of L15.end L40.end
  measures "d109" distance of L15.end L12.end
  measures "d110" distance of L15.end L40.end
  measures "d111" distance of L15.end L46.end
  measures "d112" distance of L12.end L41.end
  measures "d113" distance of L12.end L50.end
  measures "d226" distance of L8.end L7.end
  measures "d227" distance of L8.end L54.end
  measures "d228" distance of L9.end L10.end
  measures "d229" distance of L9.end L58.end
  measures "d230" distance of L14.end L15.end
  measures "d231" distance of L14.end L62.end
  measures "d232" distance of L13.end L12.end
  measures "d233" distance of L13.end L66.end
extrude "Extrude4" cut sketch "Sketch3" against normal blind 48 contours L4 L7 L8 L52 L53 L54 L55 | L4 L10 L17 L56 L57 L58 L59 | L4 L15 L60 L61 L62 L63 | L4 L8 L9 L10 L11 L17 L23 L27 L29 L35 L52 L56 | L4 L13 L14 L15 L16 L18 L19 L39 L43 L47 L51 L60 L64 | L4 L12 L13 L64 L65 L66 L67 bodies 1
extrude "Extrude9" add sketch "Sketch1" along normal blind 12 and the other way blind -6 separate body contours L56 L59 L80 L81 L82 L83 A27 | L56 L57 L59 L62 L77 L78 L81 L82 A26 A27 L93 L94 L97 L98 A30 A31 | L56 L57 L76 L77 L78 L79 A26 | L59 L62 L96 L97 L98 L99 A31 | L57 L59 L62 L63 L65 L92 L96 L102 | L57 L59 L63 L65 L100 L101 L102 L103 | L57 L62 L92 L93 L94 L95 A30 | L57 L59 L63 L64 L65 L84 L88 L100 | L59 L64 L88 L89 L90 L91 A29 | L57 L58 L59 L64 L69 L70 L73 L74 A24 A25 L85 L86 A28 L89 L90 A29 L144 | L57 L64 L84 L85 L86 L87 A28 | L58 L59 L72 L73 L74 L75 A25 L144 | L57 L58 L68 L69 L70 L71 A24 L144 makes body 2
extrude "Extrude10" cut sketch "Sketch1" along normal blind 9 contours L57 L59 L63 L65 L100 L101 L102 L103 bodies 2
extrude "Extrude11" add sketch "Sketch1" along normal blind 12 and the other way blind -8.5 separate body contours L106 L107 L109 L114 | L109 L113 L114 L116 L117 L119 L122 L126 L127 L130 | L107 L108 L112 L114 L115 L121 L124 L125 L126 L130 | L108 L109 L112 L113 L117 L119 L120 L121 L122 L123 L124 L127 makes body 3
extrude "Extrude12" add sketch "Sketch1" along normal blind 4.5 and the other way blind -8.5 contours L109 L113 L114 L116 L117 L119 L122 L126 L127 L130 | L107 L108 L112 L114 L115 L121 L124 L125 L126 L130 | L108 L109 L112 L113 L117 L119 L120 L121 L122 L123 L124 L127 bodies 3
fillet "Fillet1" radius 2.5 4 edges at (-53, 21, 8.25) (-53, 27, 8.25) (-47, 27, 8.25) (-47, 21, 8.25) on bodies 3
copy_body "CopyPasteBodies1" bodies 3 makes body 4
move_body "Move1" bodies 4 to x (1, 0, 0) y (0, 1, 0) z (0, 0, 1) at (15, 0, 0)
move_body "Move2" bodies 2 to x (1, 0, 0) y (0, 1, 0) z (0, 0, 1) at (-20, 0, 0)
chamfer "Chamfer1" distance 3 angle 55 2 edges at (-3.7293, -21.3035, 12) (-3.7293, 24.1965, 12) measured on face at (-0.0996, 33.0129, 12) measured on face at (-0.0996, 33.0129, 12) on bodies 1
chamfer "Chamfer2" distance 1 angle 45 20 edges at (-38.024, -13.3212, 8.5) (-38.9898, -7.2858, 8.5) (-38.986, -6.1969, 8.5) (-35.1002, -1.0013, 8.5) (-31.0045, -6.1233, 8.5) (-31.0122, -7.3119, 8.5) (-31.976, -13.3212, 8.5) (-32.9, -21, 8.5) (-35, -25.1, 8.5) (-37.1, -21, 8.5) (-53.024, -13.3212, 8.5) (-53.9898, -7.2858, 8.5) (-53.986, -6.1969, 8.5) (-50.1002, -1.0013, 8.5) (-46.0045, -6.1233, 8.5) (-46.0122, -7.3119, 8.5) (-46.976, -13.3212, 8.5) (-47.9, -21, 8.5) (-50, -25.1, 8.5) (-52.1, -21, 8.5) on bodies 3 4
chamfer "Chamfer3" distance 3 angle 30 4 edges at (-3.7293, 21.3035, 3) (-3.7293, -24.1965, 3) (-47.7322, 21.7322, 4.5) (-32.7322, 21.7322, 4.5) measured on face at (3.9801, 23.1483, 2) measured on face at (3.9801, -22.3517, 2) measured on face at (-49.381, 21.0028, 7) measured on face at (-34.381, 21.0028, 7) on bodies 1 3 4
extrude "Extrude13" add 1 faces at (8, 36.75, 4) along direction (0, 1, 0) blind 12 on bodies 1 bodies 1
sketch "Sketch4" plane through (0, 0, 12) normal (0, 0, 1) x (-1, 0, 0)
  circle A0 centre (0, 22.75) radius 7
  circle A1 centre (0, -22.75) radius 7
  circle A2 centre (-6.5, 6) radius 1.25
  circle A3 centre (6.5, 6) radius 1.25
  circle A4 centre (6.5, -6) radius 1.25
  circle A5 centre (-6.5, -6) radius 1.25
  line L0 (-24, -48.75) -> (24, -48.75)
  line L1 (0, -48.75) -> (0, -41)
  line L2 (11, -44.5) -> (-11, -44.5)
  line L3 (-11, -44.5) -> (-11, -37.5)
  line L4 (-11, -37.5) -> (11, -37.5)
  line L5 (11, -37.5) -> (11, -44.5)
  line L6 (11, -44.5) -> (-11, -37.5) construction
  line L7 (-11, -44.5) -> (11, -37.5) construction
  line L8 (11, -45.5) -> (-11, -45.5)
  line L9 (-11, -45.5) -> (-11, -36.5)
  line L10 (-11, -36.5) -> (11, -36.5)
  line L11 (11, -36.5) -> (11, -45.5)
  line L12 (11, -45.5) -> (-11, -36.5) construction
  line L13 (-11, -45.5) -> (11, -36.5) construction
  circle A6 centre (11, -41) radius 4.5
  circle A7 centre (11, -41) radius 3.5
  circle A8 centre (-11, -41) radius 3.5
  circle A9 centre (-11, -41) radius 4.5
  line L14 (23.926, 32.75) -> (21.963, 29.35)
  line L15 (21.963, 29.35) -> (18.037, 29.35)
  line L16 (18.037, 29.35) -> (16.074, 32.75)
  line L17 (16.074, 32.75) -> (18.037, 36.15)
  line L18 (18.037, 36.15) -> (21.963, 36.15)
  line L19 (21.963, 36.15) -> (23.926, 32.75)
  line L20 (23.926, -32.75) -> (21.963, -36.15)
  line L21 (21.963, -36.15) -> (18.037, -36.15)
  line L22 (18.037, -36.15) -> (16.074, -32.75)
  line L23 (16.074, -32.75) -> (18.037, -29.35)
  line L24 (18.037, -29.35) -> (21.963, -29.35)
  line L25 (21.963, -29.35) -> (23.926, -32.75)
  line L26 (-16.074, 32.75) -> (-18.037, 29.35)
  line L27 (-18.037, 29.35) -> (-21.963, 29.35)
  line L28 (-21.963, 29.35) -> (-23.926, 32.75)
  line L29 (-23.926, 32.75) -> (-21.963, 36.15)
  line L30 (-21.963, 36.15) -> (-18.037, 36.15)
  line L31 (-18.037, 36.15) -> (-16.074, 32.75)
  line L32 (-16.074, -32.75) -> (-18.037, -36.15)
  line L33 (-18.037, -36.15) -> (-21.963, -36.15)
  line L34 (-21.963, -36.15) -> (-23.926, -32.75)
  line L35 (-23.926, -32.75) -> (-21.963, -29.35)
  line L36 (-21.963, -29.35) -> (-18.037, -29.35)
  line L37 (-18.037, -29.35) -> (-16.074, -32.75)
  line L38 (23.926, 12.75) -> (21.963, 9.35)
  line L39 (21.963, 9.35) -> (18.037, 9.35)
  line L40 (18.037, 9.35) -> (16.074, 12.75)
  line L41 (16.074, 12.75) -> (18.037, 16.15)
  line L42 (18.037, 16.15) -> (21.963, 16.15)
  line L43 (21.963, 16.15) -> (23.926, 12.75)
  line L44 (-16.074, -12.75) -> (-18.037, -16.15)
  line L45 (-18.037, -16.15) -> (-21.963, -16.15)
  line L46 (-21.963, -16.15) -> (-23.926, -12.75)
  line L47 (-23.926, -12.75) -> (-21.963, -9.35)
  line L48 (-21.963, -9.35) -> (-18.037, -9.35)
  line L49 (-18.037, -9.35) -> (-16.074, -12.75)
  line L50 (-16.074, 12.75) -> (-18.037, 9.35)
  line L51 (-18.037, 9.35) -> (-21.963, 9.35)
  line L52 (-21.963, 9.35) -> (-23.926, 12.75)
  line L53 (-23.926, 12.75) -> (-21.963, 16.15)
  line L54 (-21.963, 16.15) -> (-18.037, 16.15)
  line L55 (-18.037, 16.15) -> (-16.074, 12.75)
  line L56 (23.926, -12.75) -> (21.963, -16.15)
  line L57 (21.963, -16.15) -> (18.037, -16.15)
  line L58 (18.037, -16.15) -> (16.074, -12.75)
  line L59 (16.074, -12.75) -> (18.037, -9.35)
  line L60 (18.037, -9.35) -> (21.963, -9.35)
  line L61 (21.963, -9.35) -> (23.926, -12.75)
  point P0 (0, -41)
  point P1 (0, -41)
  dimension "d245" = 7.75
  dimension "d246" = 22
  dimension "d247" = 7
  dimension "d248" = 22
  dimension "d249" = 9
  dimension "d250" = 9
  dimension "d251" = 7
  dimension "d252" = 7
  dimension "d253" = 9
  constraint midpoint L0 L1.start
  constraint perpendicular L0 L1
  constraint horizontal L2
  constraint perpendicular L2 L3
  constraint parallel L2 L4
  constraint parallel L3 L5
  constraint coincident L6 P1
  constraint coincident L7 P1
  constraint coincident P1 P0
  constraint horizontal L8
  constraint perpendicular L8 L9
  constraint parallel L8 L10
  constraint parallel L9 L11
  constraint coincident L12 P1
  constraint coincident L13 P1
  constraint midpoint L11 A6.centre
  constraint concentric A6 A7
  constraint midpoint L9 A8.centre
  constraint concentric A8 A9
  measures "d245" distance of L1.start P1
  measures "d246" distance of L3.end L4.end
  measures "d247" distance of L2.end L3.end
  measures "d248" distance of L9.end L10.end
  measures "d249" distance of L8.end L9.end
  measures "d250" diameter of A6
  measures "d251" diameter of A7
  measures "d252" diameter of A8
  measures "d253" diameter of A9
extrude "Extrude14" cut sketch "Sketch4" against normal blind 12 contours L1 L2 L8 A9 | L1 L2 L8 A6 | L2 L4 A6 A9 | L2 L11 A6 | L11 A6 A7 | L9 A8 A9 | L2 L9 A9 | L2 L4 A6 A7 | L2 L4 A8 A9 | L5 L11 A7 | L5 L11 A7 | L3 L9 A8 | L3 L9 A8 | L4 L9 A9 | L4 L10 A6 A9 | L4 L11 A6 bodies 1
extrude "Extrude15" add sketch "Sketch4" against normal blind 1 contours L1 L2 L8 A9 | L1 L2 L8 A6 | L2 L11 A6 | L11 A6 A7 | L9 A8 A9 | L2 L9 A9 | L4 L9 A9 | L4 L10 A6 A9 | L4 L11 A6 bodies 1
equation "d6 = d5"
equation "d7 = d5"
equation "d8 = d5"
equation "d9 = 7 mm + d42"
equation "d12 = d2 + ( 2 * d39 ) + 4 * ( d38 - d39 / 2 - 0 mm )"
equation "d31 = d30"
equation "d32 = d31"
equation "d33 = d31"
equation "d40 = d38"
equation "d41 = d39"
equation "d43 = d12"
equation "d44 = d38 - d39 / 2 - 2 mm"
equation "d46 = d39 + ( 2 * 2 ) * 1 mm"
equation "d47 = d44"
equation "d49 = d46"
equation "d51 = d50"
equation "d52 = d50"
equation "d53 = d50"
equation "d54 = d51"
equation "d55 = d51"
equation "d56 = d54"
equation "d57 = d54"
equation "d62 = d63"
equation "d63 = d64"
equation "d64 = d65"
equation "d68 = d62"
equation "d86 = d50"
equation "d87 = d50"
equation "d88 = d50"
equation "d89 = d50"
equation "d90 = d50"
equation "d91 = d50"
equation "d92 = d50"
equation "d93 = d50"
equation "d94 = d64"
equation "d95 = d64"
equation "d96 = d64"
equation "d97 = d64"
equation "d99 = d46"
equation "d101 = d99"
equation "d102 = d100"
equation "d104 = d102"
equation "d105 = d103"
equation "d106 = d98"
equation "d107 = d49"
equation "d108 = d104"
equation "d109 = d107"
equation "d110 = d108"
equation "d111 = d105"
equation "d112 = d110"
equation "d113 = d111"
equation "d114 = d38"
equation "d115 = d38"
equation "d117 = d116"
equation "d118 = d11"
equation "d119 = d12"
equation "d120 = d1"
equation "d121 = d2"
equation "d122 = d50"
equation "d123 = d50"
equation "d124 = d50"
equation "d125 = d50"
equation "d126 = d50"
equation "d127 = d50"
equation "d128 = d50"
equation "d129 = d50"
equation "d130 = d62 + 0.8 mm"
equation "d131 = d130"
equation "d132 = d130"
equation "d133 = d130"
equation "d134 = 7 mm + d42"
equation "d136 = d50"
equation "d137 = d50"
equation "d138 = d130"
equation "d139 = d50"
equation "d140 = d50"
equation "d141 = d130"
equation "d142 = d50"
equation "d143 = d50"
equation "d144 = d50"
equation "d145 = d50"
equation "d146 = d130"
equation "d147 = d130"
equation "d148 = d1"
equation "d150 = 1 mm + d42 + 3 mm"
equation "d152 = -( 7 mm + d42 ) + 6 mm"
equation "d154 = d46 + 2 mm"
equation "d155 = d157 / 2 + d162 + d164 + d165 + d168 + d11 / 2 + 2 mm - 20 mm"
equation "d156 = d154"
equation "d158 = d156 / 2"
equation "d159 = d157 / 2"
equation "d161 = d160"
equation "d162 = d1 / 2 + d157 / 2"
equation "d163 = d39"
equation "d166 = d163"
equation "d167 = d166 / 2 + 0.2 mm"
equation "d169 = d167"
equation "d170 = 7 mm + d42"
equation "d172 = -( 7 mm + d42 ) + 3.5 mm"
equation "d245 = 12 mm - 4.25 mm"
